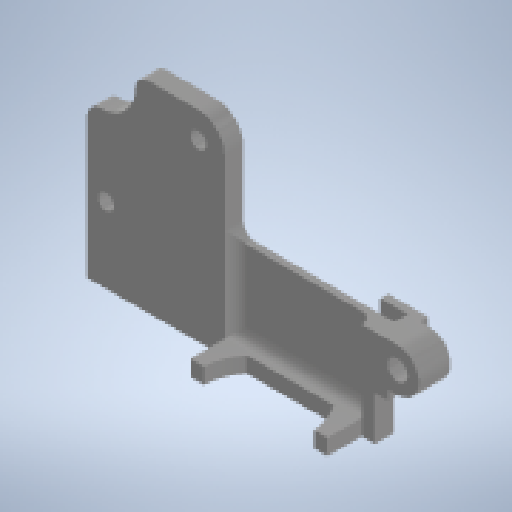
# Autodesk Inventor part: BACKPLATE
Saved by Autodesk Inventor 2023 (Build 270158000, 158)
## iProperties
Created: 2022-01-01
Part Number: BACKPLATE
Material: PET Plastic
Document SubType Name: Modeling
Designer: a laptop
Density: 1.541 g/cm^3
Appearance: Polycarbonate - Clear
Author: a laptop
Autodesk Inventor part; units mm, degrees
ref_plane "YZ Plane" through (0, 0, 0) normal (1, 0, 0) x (0, 1, 0)
ref_plane "XZ Plane" through (0, 0, 0) normal (0, 1, 0) x (-1, 0, 0)
ref_plane "XY Plane" through (0, 0, 0) normal (0, 0, 1) x (1, 0, 0)
sketch "Sketch1" plane through (0, 0, 0) normal (0, 0, 1) x (1, 0, 0)
  arc A0 (-20, 13.65) -> (-13.5, 20.15) centre (-20, 20.15) ccw
  circle A1 centre (-20, 20.15) radius 4.5 projected
  arc A2 (-20, 13.65) -> (-22.5, 11.15) centre (-20, 11.15) ccw
  line L0 (-22.5, 11.15) -> (-22.5, -15.45)
  circle A3 centre (-19, -1.2) radius 1.5 projected
  line L1 (-22.5, -15.45) -> (-15, -15.45)
  line L2 (34.5, -7.1) -> (34.5, 2.9)
  line L3 (34.5, 2.9) -> (32, 2.9)
  arc A4 (3.45, 17.7) -> (-1.5, 22.65) centre (-1.5, 17.7) ccw
  circle A5 centre (-1.5, 17.7) radius 1.5 projected
  arc A6 (-11, 22.65) -> (-13.5, 20.15) centre (-11, 20.15) ccw
  line L4 (-11, 22.65) -> (-1.5, 22.65)
  arc A7 (3.45, 5.4) -> (5.95, 2.9) centre (5.95, 5.4) ccw
  line L5 (3.45, 5.4) -> (3.45, 17.7)
  circle A8 centre (23.5, 7.6) radius 2.7 projected
  line L6 (-15, -15.45) -> (32, -15.45)
  line L7 (32, 20.05) -> (32, 2.9) construction
  line L8 (32, 2.9) -> (5.95, 2.9)
  line L9 (32, -15.45) -> (32, -7.1)
  line L10 (32, -7.1) -> (34.5, -7.1)
  point P0 (0, 0)
  point P1 (-32, -15.45)
  dimension "d0" = 90
  dimension "d1" = 90
  dimension "d2" = 2
  dimension "d3" = 3.5
  dimension "d5" = 90
  dimension "d6" = 90
  dimension "d7" = 4.7
  dimension "d51" = 2.5
  dimension "d52" = 10
  constraints: 22 end point, 10 point on circle, 8 perpendicular, 7 tangent, 5 centre point, 3 vertical, 2 concentric, 2 equal radius, 1 coincident, 1 horizontal, 1 horizontal alignment, 3 other
  measures "d2" radial gap between concentric circles of A0 A1
  measures "d3" distance from line of L0 A3.centre
  measures "d7" distance from line of L3 A8.centre
  measures "d51" horizontal distance of L2.start L3.end
  measures "d52" distance of L2.start L2.end
extrude "Extrusion1" add sketch "Sketch1" along normal blind 3.5 contours A0 A6 L4 A4 L5 A7 L8 L3 L2 L10 L9 L6 L1 L0 A2
sketch "Sketch2" plane through (0, 0, 3.5) normal (0, 0, 1) x (1, 0, 0)
  line L0 (29.5, 12.55) -> (29.5, -12.45)
  line L1 (29.5, -12.45) -> (3.5, -12.45)
  line L2 (29.5, 12.55) -> (3.5, 12.55)
  line L3 (3.5, 12.55) -> (3.5, -12.45)
  point P0 (0, 0)
  point P1 (6.5, -20.5)
  point P2 (26.5, -20.5)
  point P3 (32, -15.45)
  dimension "d14" = 3
  dimension "d15" = 3
  dimension "d16" = 25
  dimension "d53" = 2.5
  dimension "d54" = 3
  constraints: 8 end point, 3 perpendicular, 1 horizontal, 2 other
  measures "d14" distance from line of L3 point (6.5, -20.5)
  measures "d15" horizontal distance of L0.end point (26.5, -20.5)
  measures "d16" distance of L0.start L0.end
  measures "d53" horizontal distance of point (32, -15.45) L0.end
  measures "d54" vertical distance of point (32, -15.45) L0.end
extrude "Extrusion2" cut sketch "Sketch2" against normal blind 2.2
fillet "Fillet1" radius 2 3 edges at (16.5, -12.45, 1.3) (3.5, -3.7737, 1.3) (29.5, -4.775, 1.3)
sketch "Sketch3" plane through (-15, -15.45, 0) normal (0, -1, 0) x (1, 0, 0)
  circle A0 centre (31.5, 10.5) radius 4.3 construction
  line L0 (39.5, 4.5) -> (23.5, 4.5) projected
  arc A1 (39.5, 4.5) -> (39.5, 16.5) centre (31.5, 10.5) ccw projected
  line L1 (23.5, 16.5) -> (39.5, 16.5) projected
  arc A2 (23.5, 16.5) -> (23.5, 4.5) centre (31.5, 10.5) ccw projected
  line L2 (39.6976, 16.9) -> (23.3024, 16.9) construction
  line L3 (39.6976, 4.1) -> (23.3024, 4.1)
  arc A3 (39.6976, 4.1) -> (41.888, 10) centre (31.5, 10.5) ccw
  arc A4 (23.3024, 16.9) -> (21.1, 10.5) centre (31.5, 10.5) ccw construction
  line L4 (41.9, 3.5) -> (21.1, 3.5)
  line L5 (21.1, 3.5) -> (21.1, 10.5) construction
  line L6 (41.9, 3.5) -> (41.9, 10.5) construction
  arc A5 (41.9, 10.5) -> (39.6976, 16.9) centre (31.5, 10.5) ccw construction
  arc A6 (21.1, 10.5) -> (21.112, 10) centre (31.5, 10.5) ccw construction
  line L7 (21.1, 10.5) -> (18.5, 10.5) construction
  line L8 (18.5, 10.5) -> (18.5, 10) construction
  line L9 (18.5, 3.5) -> (21.1, 3.5)
  line L10 (41.9, 10.5) -> (44.5, 10.5) construction
  line L11 (44.5, 10.5) -> (44.5, 10) construction
  line L12 (44.5, 3.5) -> (41.9, 3.5)
  line L13 (21.112, 10) -> (18.5, 10)
  line L14 (18.5, 10) -> (18.5, 3.5)
  arc A7 (21.112, 10) -> (23.3024, 4.1) centre (31.5, 10.5) ccw
  line L15 (41.888, 10) -> (44.5, 10)
  arc A8 (41.888, 10) -> (41.9, 10.5) centre (31.5, 10.5) ccw construction
  line L16 (44.5, 10) -> (44.5, 3.5)
  point P0 (15, 0)
  point P1 (19.806, 10)
  point P2 (43.194, 10)
  dimension "d22" = 0.4
  dimension "d23" = 0.4
  dimension "d55" = 6.5
  constraints: 30 end point, 14 perpendicular, 12 point on circle, 6 centre point, 3 coincident, 3 horizontal, 2 equal length, 2 midpoint, 2 tangent, 2 vertical, 1 concentric, 1 horizontal alignment, 1 parallel, 1 vertical alignment
  measures "d22" distance between parallel lines of L1 L2
  measures "d23" radial gap between concentric circles of A1 A3
  measures "d55" distance between parallel lines of L12 L15
extrude "Extrusion3" add sketch "Sketch3" against normal blind 3 contours A3 L15 L16 L12 L4 L9 L14 L13 A7 L3
sketch "Sketch4" plane through (0, 0, 0) normal (0, 0, -1) x (-1, 0, 0)
  line L0 (-32, -15.45) -> (-32, 20.05) projected
  line L1 (-34.5, -7.1) -> (-34.5, 2.9) projected
  line L2 (22.5, 11.15) -> (22.5, -15.45) projected
  arc A0 (22.5, 11.15) -> (20, 13.65) centre (20, 11.15) ccw projected
  arc A1 (13.5, 20.15) -> (20, 13.65) centre (20, 20.15) ccw projected
  arc A2 (13.5, 20.15) -> (11, 22.65) centre (11, 20.15) ccw projected
  line L3 (1.5, 22.65) -> (11, 22.65) projected
  arc A3 (1.5, 22.65) -> (-3.45, 17.7) centre (1.5, 17.7) ccw projected
  line L4 (-3.45, 5.4) -> (-3.45, 17.7) projected
  arc A4 (-5.95, 2.9) -> (-3.45, 5.4) centre (-5.95, 5.4) ccw projected
  line L5 (-34.5, 2.9) -> (-5.95, 2.9) projected
  line L6 (-34.5, -7.1) -> (-34.5, 2.9) projected
  line L7 (-32, -7.1) -> (-34.5, -7.1) projected
  line L8 (-32, -15.45) -> (-32, -7.1) projected
  line L9 (22.5, -15.45) -> (-32, -15.45) projected
  circle A5 centre (19, -1.2) radius 1.5 projected
  circle A6 centre (1.5, 17.7) radius 1.5 projected
  line L10 (-32, -7.1) -> (-34.5, -7.1) projected
  point P0 (0, 0)
  point P1 (-32, 2.9)
extrude "Extrusion4" add sketch "Sketch4" along normal blind 4.05 contours L7 L1 L5 L0
sketch "Sketch5" plane through (32, -15.45, 0) normal (-1, 0, 0) x (0, 0, 1)
  line L0 (-4.05, 18.35) -> (-2.55, 18.35)
  line L1 (-2.55, 18.35) -> (-2.55, 8.35)
  line L2 (-2.55, 8.35) -> (-4.05, 8.35)
  line L3 (-4.05, 8.35) -> (-4.05, 18.35)
  point P0 (0, 15.45)
  dimension "d57" = 1.5
  constraints: 8 end point, 2 coincident, 2 parallel, 1 horizontal, 1 perpendicular
  measures "d57" distance of L0.start L0.end
extrude "Extrusion5" add sketch "Sketch5" along normal blind 5
sketch "Sketch8" plane through (0, 0, 3.5) normal (0, 0, 1) x (1, 0, 0)
  circle A0 centre (36.25, -1.2) radius 1.7
  arc A1 (36.25, -5.3) -> (36.25, 2.9) centre (36.25, -1.2) ccw
  line L0 (36.25, 2.9) -> (34.5, 2.9)
  line L1 (36.25, -5.3) -> (34.5, -5.3)
  arc A2 (34.5, 2.9) -> (34.5, -5.3) centre (36.25, -1.2) ccw
  point P0 (0, 0)
  dimension "d35" = 3.4
  dimension "d36" = 2.4
  dimension "d37" = 1.75
  constraints: 4 end point, 4 point on circle, 3 centre point, 2 concentric, 2 vertical alignment, 1 horizontal, 1 parallel
  measures "d35" diameter of A0
  measures "d36" radial gap between concentric circles of A1 A0
  measures "d37" distance of L0.start L0.end
extrude "Extrusion7" add sketch "Sketch8" against normal blind 6
sketch "Sketch9" plane through (0, 0, -2.5) normal (0, 0, -1) x (-1, 0, 0)
  line L0 (-34.6046, -4.05) -> (-37.8954, -4.05)
  line L1 (-37.8954, -4.05) -> (-39.5409, -1.2)
  line L2 (-39.5409, -1.2) -> (-37.8954, 1.65)
  line L3 (-37.8954, 1.65) -> (-34.6046, 1.65)
  line L4 (-34.6046, 1.65) -> (-32.9591, -1.2)
  line L5 (-32.9591, -1.2) -> (-34.6046, -4.05)
  circle A0 centre (-36.25, -1.2) radius 1.7 projected
  point P0 (0, 0)
  point P1 (-36.25, -1.2)
  point P2 (-34.5, -2.718)
  point P3 (-34.5, -0.482)
  point P4 (-34.5, -0.4601)
  point P5 (-34.5, -1.9399)
  dimension "d42" = 5.7
  constraints: 12 end point, 1 coincident, 1 horizontal, 14 other
  measures "d42" distance between parallel lines of L0 L3
extrude "Extrusion9" cut sketch "Sketch9" along normal blind 6 and the other way blind 3 contours L0 L1 L2 L3 L4 L5 | A0
sketch "Sketch10" plane through (5.95, 2.9, 1.3) normal (0, 1, 0) x (1, 0, 0)
  line L0 (26.05, 3.8) -> (26.05, 1.3) projected
  line L1 (26.2, 1.3) -> (26.2, 3.8)
  line L2 (26.2, 3.8) -> (26.05, 3.8)
  line L3 (26.05, 1.3) -> (26.2, 1.3)
  point P0 (-5.95, 1.3)
  dimension "d47" = 0.15
  constraints: 6 end point, 2 perpendicular, 1 point on line, 1 vertical
  measures "d47" distance between parallel lines of L0 L1
extrude "Extrusion10" cut sketch "Sketch10" against normal blind 10
body "Solid1"
